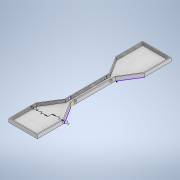
# Autodesk Inventor part: Ant_Project
Saved by Autodesk Inventor 2020 (Build 240168000, 168)
## iProperties
Created: 2019-10-17
Part Number: Ant_Project
Material: Generic
Document SubType Name: Modeling
Designer: cks4a449
Density: 1 g/cm^3
Appearance: Default
Author: cks4a449
## iProperties of the stored document _3DPrint.ipt
Created: 2019-10-17
Part Number: _3DPrint
Material: Generic
Document SubType Name: Modeling
Designer: cks4a449
Density: 1 g/cm^3
Appearance: Default
Author: cks4a449
Autodesk Inventor part; units mm, degrees
ref_plane "YZ Plane" through (0, 0, 0) normal (1, 0, 0) x (0, 1, 0)
ref_plane "XZ Plane" through (0, 0, 0) normal (0, 1, 0) x (-1, 0, 0)
ref_plane "XY Plane" through (0, 0, 0) normal (0, 0, 1) x (1, 0, 0)
sketch "Sketch1" plane through (0, 0, 0) normal (0, 1, 0) x (-1, 0, 0)
  line L0 (0, 0) -> (20, 0)
  line L1 (10, -100) -> (15, -100)
  line L2 (10, -100) -> (5, -100)
  line L3 (15, -100) -> (15, 0)
  line L4 (5, -100) -> (5, 0)
  line L5 (15, -100) -> (17, -100)
  line L6 (17, -100) -> (17, 0)
  line L7 (5, -100) -> (3, -100)
  line L8 (3, -100) -> (3, 0.3155)
  point P0 (3, 0)
  dimension "d2" = 5
  dimension "d3" = 5
  dimension "d4" = 2
  dimension "d5" = 2
  constraints: 18 end point, 4 perpendicular, 3 horizontal, 3 point on line
  measures "d2" distance of L1.start L1.end
  measures "d3" distance of L1.start L2.end
  measures "d4" distance of L1.end L5.end
  measures "d5" distance of L2.end L7.end
extrude "Extrusion1" add sketch "Sketch1" along normal blind 2 contours L0 L3 L1 L2 L4
extrude "Extrusion2" add sketch "Sketch1" along normal blind 8 contours L4 L7 L8 L0 | L0 L6 L5 L3
sketch "Sketch2" plane through (-3, 0, 0) normal (1, 0, 0) x (0, 0, -1)
  line L0 (0, 2) -> (0, 8) projected
  line L1 (100, 0) -> (100, 8) projected
  line L2 (50, 5) -> (10, 5)
  line L3 (50, 5) -> (90, 5)
  circle A0 centre (10, 5) radius 3
  circle A1 centre (90, 5) radius 3
  point P0 (0, 0)
  dimension "d10" = 40
  dimension "d12" = 6
  dimension "d13" = 6
  constraints: 4 end point, 2 centre point, 2 coincident
  measures "d10" distance of L2.start L2.end
  measures "d12" diameter of A0
  measures "d13" diameter of A1
extrude "Extrusion3" cut sketch "Sketch2" against normal blind 8
sketch "Sketch3" plane through (-17, 0, -100) normal (-1, 0, 0) x (0, 0, 1)
  line L0 (100, 2) -> (100, 8) projected
  line L1 (0, 2) -> (0, 8) projected
  line L2 (50, 5) -> (90, 5)
  line L3 (50, 5) -> (10, 5)
  line L4 (10, 5) -> (13, 5)
  line L5 (10, 7.5) -> (12, 7.5)
  line L6 (10, 7.5) -> (8, 7.5)
  line L7 (10, 2.5) -> (12, 2.5)
  line L8 (10, 2.5) -> (8, 2.5)
  line L9 (7, 5) -> (7, 6)
  line L10 (7, 5) -> (7, 4)
  line L11 (13, 5) -> (13, 6)
  line L12 (13, 5) -> (13, 4)
  arc A0 (12, 2.5) -> (13, 4) centre (11.375, 4) ccw
  arc A1 (7, 4) -> (8, 2.5) centre (8.625, 4) ccw
  arc A2 (13, 6) -> (12, 7.5) centre (11.375, 6) ccw
  arc A3 (8, 7.5) -> (7, 6) centre (8.625, 6) ccw
  line L13 (50, 5) -> (50, 8)
  line L14 (0, 8) -> (100, 8) projected
  line L15 (90, 7.5) -> (88, 7.5)
  line L16 (90, 7.5) -> (92, 7.5)
  line L17 (90, 2.5) -> (88, 2.5)
  line L18 (90, 2.5) -> (92, 2.5)
  line L19 (93, 5) -> (93, 6)
  line L20 (93, 5) -> (93, 4)
  line L21 (87, 5) -> (87, 6)
  line L22 (87, 5) -> (87, 4)
  arc A4 (87, 4) -> (88, 2.5) centre (88.625, 4) ccw
  arc A5 (92, 2.5) -> (93, 4) centre (91.375, 4) ccw
  arc A6 (88, 7.5) -> (87, 6) centre (88.625, 6) ccw
  arc A7 (93, 6) -> (92, 7.5) centre (91.375, 6) ccw
  point P0 (100, 0)
  dimension "d25" = 2
  constraints: 40 end point, 16 point on circle, 16 symmetric about line, 8 centre point, 4 tangent, 4 vertical, 3 horizontal, 1 midpoint, 1 point on line, 4 other
  measures "d25" distance of L7.start L8.end
extrude "Extrusion4" cut sketch "Sketch3" against normal blind 8
sketch "Sketch4" plane through (0, 0, 0) normal (0, 1, 0) x (-1, 0, 0)
  line L0 (17, 0) -> (3, 0) projected
  line L1 (10, 0) -> (10, 40)
  line L2 (10, 40) -> (-20, 40)
  line L3 (10, 40) -> (40, 40)
  line L4 (40, 40) -> (15, 0)
  line L5 (15, 0) -> (4.9463, 0)
  line L6 (-20, 40) -> (4.9463, 0)
  line L7 (40, 40) -> (42, 40)
  line L8 (42, 40) -> (17, 0)
  line L9 (-20, 40) -> (-22, 40)
  line L10 (-22, 40) -> (3, 0)
  line L11 (17, -100) -> (17, 0) projected
  line L12 (17, -50) -> (3, -50)
  line L13 (17, -100) -> (3, -100)
  line L14 (10, -100) -> (10, -140)
  line L15 (10, -140) -> (-20, -140)
  line L16 (10, -140) -> (40, -140)
  line L17 (40, -140) -> (15, -100)
  line L18 (15, -100) -> (4.9463, -100)
  line L19 (-20, -140) -> (4.9463, -100)
  line L20 (40, -140) -> (42, -140)
  line L21 (42, -140) -> (17, -100)
  line L22 (-20, -140) -> (-22, -140)
  line L23 (-22, -140) -> (3, -100)
  line L24 (17, 0) -> (17, -100)
  point P0 (0, 0)
  point P1 (0, -100)
  dimension "d35" = 30
  dimension "d36" = 30
  dimension "d37" = 2
  dimension "d38" = 2
  constraints: 46 end point, 13 symmetric about line, 5 horizontal, 2 midpoint, 2 point on line, 1 vertical
  measures "d35" distance of L1.end L2.end
  measures "d36" distance of L1.end L3.end
  measures "d37" distance of L7.start L7.end
  measures "d38" distance of L2.end L9.end
extrude "Extrusion5" add sketch "Sketch4" along normal blind 2 contours L0 L1 L3 L4 | L0 L6 L2 L1
extrude "Extrusion6" add sketch "Sketch4" along normal blind 8 contours L0 L4 L7 L8 | L0 L10 L9 L6
sketch "Sketch5" plane through (-42, 0, 40) normal (0, 0, 1) x (1, 0, 0)
  line L0 (0, 0) -> (0, 8) projected
  line L1 (0, 0) -> (64, 0) projected
  line L2 (0, 0) -> (64, 0)
  line L3 (64, 0) -> (64, 8) projected
  line L4 (64, 0) -> (64, 8)
  line L5 (37.0537, 8) -> (62, 8) projected
  line L6 (64, 8) -> (62, 8)
  line L7 (62, 2) -> (62, 8) projected
  line L8 (62, 8) -> (62, 2)
  line L9 (2, 2) -> (2, 8) projected
  line L10 (62, 2) -> (2, 2)
  line L11 (2, 2) -> (2, 8)
  line L12 (2, 8) -> (0, 8)
  line L13 (0, 8) -> (0, 0)
  point P0 (42, 0)
  constraints: 16 end point, 4 perpendicular, 2 collinear, 1 horizontal, 1 point on line
extrude "Extrusion7" add sketch "Sketch5" along normal blind 60
extrude "Extrusion8" add sketch "Sketch4" along normal blind 2 contours L17 L16 L14 L13 | L14 L15 L19 L13
extrude "Extrusion9" add sketch "Sketch4" along normal blind 8 contours L21 L20 L17 L13 | L19 L22 L23 L13
sketch "Sketch6" plane through (22, 0, -140) normal (0, 0, -1) x (-1, 0, 0)
  line L0 (0, 8) -> (2, 8) projected
  line L1 (0, 0) -> (0, 8) projected
  line L2 (0, 8) -> (0, 0)
  line L3 (64, 8) -> (64, 0) projected
  line L4 (0, 0) -> (64, 0)
  line L5 (64, 0) -> (64, 8)
  line L6 (62, 8) -> (37, 8) projected
  line L7 (64, 8) -> (62, 8)
  line L8 (62, 2) -> (62, 8) projected
  line L9 (62, 8) -> (62, 2)
  line L10 (2, 2) -> (62, 2) projected
  line L11 (62, 2) -> (2, 2)
  line L12 (2, 8) -> (2, 2) projected
  line L13 (2, 2) -> (2, 8)
  line L14 (2, 8) -> (0, 8)
  point P0 (22, 0)
  constraints: 16 end point, 5 collinear, 3 perpendicular
extrude "Extrusion10" add sketch "Sketch6" along normal blind 60
sketch "Sketch7" plane through (0, 2, 0) normal (0, 1, 0) x (1, 0, 0)
  point P0 (0, 0)
sketch "Sketch8" plane through (0, 2, 0) normal (0, 1, 0) x (1, 0, 0)
  line L0 (-40, -40) -> (-40, -100) projected
  line L1 (20, -40) -> (20, -100) projected
  line L2 (-40, -100) -> (20, -100)
  line L3 (20, -100) -> (20, -98)
  line L4 (20, -98) -> (-40, -98)
  line L5 (-40, -98) -> (-40, -100)
  line L6 (-40, 200) -> (20, 200) projected
  line L7 (-40, 200) -> (20, 200)
  line L8 (20, 200) -> (20, 198)
  line L9 (20, 198) -> (-40, 198)
  line L10 (-40, 198) -> (-40, 200)
  point P0 (0, 0)
  dimension "d51" = 2
  dimension "d52" = 60
  dimension "d53" = 2
  constraints: 16 end point, 4 parallel, 2 horizontal, 2 perpendicular, 1 point on line
  measures "d51" distance of L3.end L2.end
  measures "d52" distance of L8.end L9.end
  measures "d53" distance of L7.end L8.end
extrude "Extrusion11" add sketch "Sketch8" along normal blind 6
body "Solid1"
